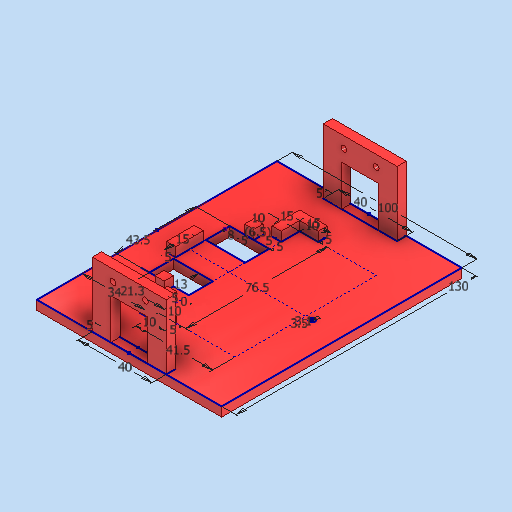
# Autodesk Inventor part: Chasis 1
Saved by Autodesk Inventor 2026.2 (Build 302298010, 298A)
## iProperties
Created: 2025-12-05
Part Number: Chasis 1
Material: Generic
Document SubType Name: Modeling
Designer: maxim
Density: 1 g/cm^3
Appearance: Light Red
Author: maxim
Autodesk Inventor part; units mm, degrees
ref_plane "YZ Plane" through (0, 0, 0) normal (1, 0, 0) x (0, 1, 0)
ref_plane "XZ Plane" through (0, 0, 0) normal (0, 1, 0) x (-1, 0, 0)
ref_plane "XY Plane" through (0, 0, 0) normal (0, 0, 1) x (1, 0, 0)
sketch "Sketch1" plane through (0, 0, 0) normal (0, 1, 0) x (-1, 0, 0)
  line L0 (0, 0) -> (100, 0)
  line L1 (100, 0) -> (100, -130)
  line L2 (100, -130) -> (0, -130)
  line L3 (0, -130) -> (0, 0)
  line L4 (61, -26.75) -> (19.5, -26.75) construction
  line L5 (19.5, -26.75) -> (19.5, -103.25) construction
  line L6 (19.5, -103.25) -> (61, -103.25) construction
  line L7 (61, -103.25) -> (61, -26.75) construction
  line L8 (61, -65) -> (19.5, -65) construction
  line L9 (70, 0) -> (30, 0)
  line L10 (30, 0) -> (30, -5)
  line L11 (30, -5) -> (70, -5)
  line L12 (70, -5) -> (70, 0)
  line L13 (70, -130) -> (30, -130)
  line L14 (30, -130) -> (30, -125)
  line L15 (30, -125) -> (70, -125)
  line L16 (70, -125) -> (70, -130)
  line L17 (61, -26.75) -> (51, -26.75)
  line L18 (51, -21.75) -> (66, -21.75)
  line L19 (66, -21.75) -> (66, -36.75)
  line L20 (66, -36.75) -> (61, -36.75)
  line L21 (61, -26.75) -> (61, -36.75)
  line L22 (51, -103.25) -> (51, -108.25)
  line L23 (51, -108.25) -> (66, -108.25)
  line L24 (66, -108.25) -> (66, -93.25)
  line L25 (66, -93.25) -> (61, -93.25)
  line L26 (61, -103.25) -> (61, -93.25)
  line L27 (61, -103.25) -> (51, -103.25)
  line L28 (82.3, -43.25) -> (61, -43.25) construction
  line L29 (61, -43.25) -> (61, -86.75) construction
  line L30 (61, -86.75) -> (82.3, -86.75) construction
  line L31 (82.3, -86.75) -> (82.3, -43.25) construction
  line L32 (82.3, -43.25) -> (82.3, -48.25)
  line L33 (87.05, -43.25) -> (82.3, -43.25)
  line L34 (82.3, -43.25) -> (61, -43.25)
  line L35 (61, -43.25) -> (61, -56.25)
  line L36 (61, -56.25) -> (82.3, -56.25)
  line L37 (82.3, -56.25) -> (82.3, -43.25)
  line L38 (82.3, -65) -> (61, -65) construction
  line L39 (82.3, -86.75) -> (61, -86.75)
  line L40 (61, -73.75) -> (82.3, -73.75)
  line L41 (82.3, -81.75) -> (82.3, -86.75)
  line L42 (61, -73.75) -> (61, -86.75)
  line L43 (51, -26.75) -> (51, -21.75)
  circle A0 centre (16, -65) radius 1.55
  line L44 (82.3, -73.75) -> (82.3, -81.75)
  line L45 (82.3, -72.5) -> (87.3, -72.5)
  line L46 (87.3, -72.5) -> (87.3, -57.5)
  line L47 (87.3, -57.5) -> (82.3, -57.5)
  line L48 (82.3, -57.5) -> (82.3, -72.5)
  line L49 (74.3, -86.75) -> (69.3, -86.75)
  line L50 (69.3, -86.75) -> (69.3, -91.75)
  line L51 (69.3, -91.75) -> (74.3, -91.75)
  line L52 (74.3, -91.75) -> (74.3, -86.75)
  line L53 (74.3, -43.25) -> (69.3, -43.25)
  line L54 (69.3, -43.25) -> (69.3, -38.25)
  line L55 (69.3, -38.25) -> (74.3, -38.25)
  line L56 (74.3, -38.25) -> (74.3, -43.25)
  point P0 (100, -65)
  point P1 (50, 0)
  point P2 (50, -5)
  point P3 (50, 0)
  point P4 (60, -115)
  point P5 (70, -115)
  point P6 (66, -29.25)
  point P7 (92.05, -81.75)
  point P8 (92.05, -48.25)
  point P9 (51, -105.75)
  point P10 (63.5, -93.25)
  point P11 (87.3, -65)
  point P12 (82.3, -84.25)
  point P13 (74.3, -89.25)
  point P14 (87.05, -43.25)
  point P15 (50, -130)
  point P16 (70, -2.5)
  point P17 (70, -127.5)
  dimension "d0" = 100
  dimension "d1" = 130
  dimension "d2" = 76.5
  dimension "d3" = 41.5
  dimension "d19" = 40
  dimension "d20" = 5
  dimension "d43" = 43.5
  dimension "d44" = 21.3
  dimension "d50" = 0
  dimension "d55" = 13
  dimension "d58" = 10
  dimension "d59" = 5
  dimension "d60" = 5
  dimension "d62" = 10
  dimension "d63" = 5
  dimension "d64" = 15
  dimension "d65" = 15
  dimension "d66" = 5
  dimension "d67" = 10
  dimension "d68" = 10
  dimension "d83" = 3.1
  dimension "d84" = 3.5
  dimension "d85" = 6.5
  dimension "d86" = 15
  dimension "d87" = 5
  dimension "d88" = 5
  dimension "d89" = 5
  dimension "d90" = 8
  dimension "d93" = 40
  dimension "d94" = 5
  dimension "d95" = 34
  constraints: 114 end point, 18 midpoint, 14 parallel, 11 horizontal, 8 perpendicular, 8 symmetric about line, 6 vertical, 5 horizontal alignment, 5 point on line, 2 collinear, 1 centre point, 1 vertical alignment
  measures "d0" distance of L1.end L2.end
  measures "d1" distance of L2.end L0.start
  measures "d2" distance of L6.end L4.start
  measures "d3" distance of L4.start L4.end
  measures "d19" distance between parallel lines of L10 L12
  measures "d20" distance between parallel lines of L11 L9
  measures "d43" distance of L30.end L28.start
  measures "d44" distance of L28.start L28.end
  measures "d50" distance between parallel lines of L29 L7
  measures "d55" distance between parallel lines of L36 L34
  measures "d58" distance between parallel lines of L20 L4
  measures "d59" distance between parallel lines of L4 L18
  measures "d60" distance between parallel lines of L7 L19
  measures "d62" distance between parallel lines of L7 L43
  measures "d63" distance of L22.start L22.end
  measures "d64" distance of L22.end L23.end
  measures "d65" distance of L23.end L25.start
  measures "d66" distance of L25.start L25.end
  measures "d67" distance from line of L7 point (51, -105.75)
  measures "d68" distance from line of point (63.5, -93.25) L6
  measures "d83" diameter of A0
  measures "d84" distance of L8.end A0.centre
  measures "d85" distance between parallel lines of L39 L25
  measures "d86" distance of L45.end L46.end
  measures "d87" distance of L46.end L47.end
  measures "d88" distance of L49.end L50.end
  measures "d89" distance between parallel lines of L50 L52
  measures "d90" horizontal distance of point (82.3, -84.25) point (74.3, -89.25)
  measures "d93" distance of L15.start L16.start
  measures "d94" distance of L16.start L13.start
  measures "d95" distance between parallel lines of L1 L19
extrude "Extrusion2" add sketch "Sketch1" against normal blind 5 contours L0 L10 L11 L12 L1 L2 L16 L15 L14 L3 | L0 L12 L11 L10 | L14 L15 L16 L2 | L17 L43 L18 L19 L20 L21 | L27 L26 L25 L24 L23 L22 | L32 L37 L36 L35 L34 | L34 L54 L55 L56 | L39 L42 L40 L44 L41 | L52 L51 L50 L39 | A0 | L48 L47 L46 L45
extrude "Extrusion3" add sketch "Sketch1" along normal blind 35 contours L0 L12 L11 L10 | L14 L15 L16 L2
sketch "Sketch2" plane through (-100, -5, 0) normal (0, 0, 1) x (1, 0, 0)
  line L0 (30, 5) -> (70, 5) projected
  line L1 (40, 5) -> (60, 5)
  line L2 (60, 5) -> (60, 27)
  line L3 (60, 27) -> (40, 27)
  line L4 (40, 27) -> (40, 5)
  line L5 (41.25, 34) -> (58.75, 34) construction
  line L6 (30, 40) -> (70, 40) projected
  point P0 (100, 5)
  point P1 (50, 5)
  point P2 (50, 27)
  point P3 (50, 34)
  dimension "d31" = 20
  dimension "d34" = 7
  dimension "d42" = 17.5
  dimension "d92" = 13
  constraints: 10 end point, 3 midpoint, 2 horizontal, 2 parallel, 2 vertical alignment, 1 horizontal alignment, 1 perpendicular, 1 point on line
  measures "d31" distance between parallel lines of L2 L4
  measures "d34" distance from line of L3 L5.start
  measures "d42" distance of L5.end L5.start
  measures "d92" distance between parallel lines of L6 L3
extrude "Extrusion6" cut sketch "Sketch2" against normal through all
hole "Hole2" at (-58.75, 29, 0) at (-41.25, 29, 0) direction (0, 0, -1) diameter 3.1 end through all
extrude "Extrusion7" cut sketch "Sketch1" against normal through all contours L32 L37 L36 L35 L34 | L39 L42 L40 L44 L41 | A0
extrude "Extrusion9" add sketch "Sketch1" along normal blind 5 contours L17 L43 L18 L19 L20 L21 | L27 L26 L25 L24 L23 L22 | L34 L54 L55 L56 | L52 L51 L50 L39 | L48 L47 L46 L45
body "Solid1"
